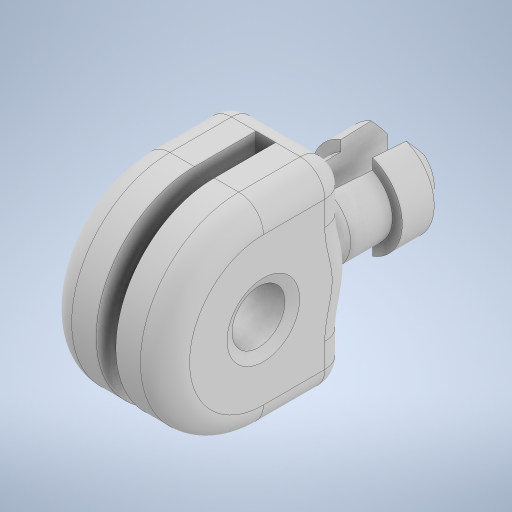
# Autodesk Inventor part: flipper_robot_v2_servo_flipper_adapter
Saved by Autodesk Inventor 2023.1 (Build 271208000, 208)
## iProperties
Created: 2025-10-28
Part Number: flipper_robot_v2_servo_flipper_adapter
Material: Generic
Document SubType Name: Modeling
Designer: Lars
Density: 1 g/cm^3
Appearance: Default
Author: Lars
Autodesk Inventor part; units mm, degrees
ref_plane "YZ Plane" through (0, 0, 0) normal (1, 0, 0) x (0, 1, 0)
ref_plane "XZ Plane" through (0, 0, 0) normal (0, 1, 0) x (-1, 0, 0)
sketch "Base Profile" plane through (0, 0, 0) normal (1, 0, 0) x (0, 1, 0)
  arc A0 (4, 0) -> (-4, 0) centre (0, 0) ccw
  line L0 (4, 0) -> (-4, 0) construction
  line L1 (-4, 0) -> (-4, -3.5)
  line L2 (-4, -3.5) -> (4, -3.5)
  line L3 (4, -3.5) -> (4, 0)
  circle A1 centre (0, 0) radius 1.075
  dimension "d0" = 8
  dimension "d1" = 3.5
  dimension "d2" = 2.15
  constraints: 8 end point, 2 centre point, 2 coincident, 2 parallel, 2 point on circle, 2 tangent, 1 horizontal, 1 perpendicular
  measures "d0" diameter of A0
  measures "d1" distance of L2.end L0.start
  measures "d2" diameter of A1
extrude "Clip Base" add sketch "Base Profile" along normal blind 4.8
ref_plane "Work Plane (Slot Cut)" through (0, 0, 4) normal (0, 0, -1) x (-1, 0, 0)
sketch "Fin Slot Layout" plane through (0, 0, 4) normal (0, 0, -1) x (-1, 0, 0)
  line L0 (0, -4) -> (-4.8, -4) projected
  line L1 (0, 4) -> (-4.8, 4) projected
  line L2 (-2.8, -4) -> (-2, -4)
  line L3 (-2, -4) -> (-2, 4)
  line L4 (-2, 4) -> (-2.8, 4)
  line L5 (-2.8, 4) -> (-2.8, -4)
  point P0 (0, 0)
  point P1 (-2.4, -4)
  dimension "d8" = 0.8
  constraints: 8 end point, 2 midpoint, 2 parallel, 2 point on line, 1 horizontal, 1 perpendicular
  measures "d8" distance between parallel lines of L3 L5
extrude "Fin Slot Cut" cut sketch "Fin Slot Layout" along normal blind 6.5
sketch "Shaft Profile" plane through (0, -4, -3.5) normal (0, 0, -1) x (-1, 0, 0)
  line L0 (0, 0) -> (0, 8) construction
  line L1 (0, 8) -> (-4.8, 8) construction
  line L2 (-4.8, 0) -> (-4.8, 8) construction
  line L3 (0, 0) -> (-4.8, 0) construction
  circle A0 centre (-2.4, 4) radius 1.45
  line L4 (-2.4, 8) -> (-2.4, 0) construction
  point P0 (0, 4)
  point P1 (-2.4, 4)
  dimension "d11" = 2.9
  constraints: 3 midpoint, 2 end point, 1 centre point, 1 coincident, 1 vertical
  measures "d11" diameter of A0
extrude "Snap Shaft" add sketch "Shaft Profile" along normal blind 4.7
sketch "Lip Profile" plane through (2.4, 0, -8.2) normal (0, 0, -1) x (-1, 0, 0)
  circle A0 centre (0, 0) radius 1.45 projected
  circle A1 centre (0, 0) radius 1.85
  point P0 (2.4, 0)
  dimension "d14" = 3.7
  constraints: 1 centre point, 1 coincident
  measures "d14" diameter of A1
extrude "Snap Lip" add sketch "Lip Profile" against normal blind 2
sketch "Upper Flex Profile" plane through (2.4, 0, -8.2) normal (0, 0, -1) x (-1, 0, 0)
  circle A0 centre (0, 0) radius 1.85 construction
  line L0 (-0.75, 1.85) -> (0.75, 1.85)
  line L1 (0.75, 1.85) -> (0.75, -1.85)
  line L2 (0.75, -1.85) -> (-0.75, -1.85)
  line L3 (-0.75, -1.85) -> (-0.75, 1.85)
  point P0 (2.4, 0)
  point P1 (0, 1.85)
  point P2 (0, -1.85)
  dimension "d18" = 1.5
  constraints: 8 end point, 2 midpoint, 2 parallel, 2 point on circle, 1 horizontal, 1 perpendicular, 1 tangent
  measures "d18" distance of L1.end L2.end
sketch "Lower Flex Profile" plane through (0, -4, -3.5) normal (0, 0, -1) x (-1, 0, 0)
  line L0 (-3.15, 5.85) -> (-1.65, 5.85) construction
  line L1 (-3.15, 2.15) -> (-3.15, 5.85) construction
  line L2 (-1.65, 2.15) -> (-3.15, 2.15) construction
  line L3 (-1.65, 5.85) -> (-1.65, 2.15) construction
  line L4 (-2.9, 5.875) -> (-1.9, 5.875)
  line L5 (-1.9, 5.875) -> (-1.9, 2.125)
  line L6 (-1.9, 2.125) -> (-2.9, 2.125)
  line L7 (-2.9, 2.125) -> (-2.9, 5.875)
  line L8 (-2.4, 2.125) -> (-2.4, 5.875) construction
  point P0 (0, 4)
  point P1 (-2.4, 4)
  point P2 (-2.4, 4)
  dimension "d20" = 1
  dimension "d21" = 3.75
  constraints: 10 end point, 3 midpoint, 2 parallel, 1 coincident, 1 horizontal, 1 perpendicular
  measures "d20" distance between parallel lines of L5 L7
  measures "d21" distance of L6.end L4.start
loft "Snap Flex Cut" cut profiles "Upper Flex Profile", "Lower Flex Profile"
chamfer "Entry Chamfer (Snap Tip)" distance 0.7 angle 45 2 edges at (4.25, 0, -8.2) (0.55, 0, -8.2)
fillet "Body Fillets (Clip Base)" radius 1 12 edges at (3.85, 0, -3.5) (0.95, 0, -3.5) (0, 0, -3.5) (4.8, 0, -3.5) (2.4, -4, -3.5) (2.4, 4, -3.5) (4.8, -4, -1.75) (4.8, 4, -1.75) (4.8, 0, 4) (0, -4, -1.75) (0, 4, -1.75) (0, 0, 4)
sketch "Hex Slot Profile" plane through (0, 0, 0) normal (-1, 0, 0) x (0, 0, 1)
  line L0 (-1.175, 2.0352) -> (1.175, 2.0352)
  line L1 (1.175, 2.0352) -> (2.35, 0)
  line L2 (2.35, 0) -> (1.175, -2.0352)
  line L3 (1.175, -2.0352) -> (-1.175, -2.0352)
  line L4 (-1.175, -2.0352) -> (-2.35, 0)
  line L5 (-2.35, 0) -> (-1.175, 2.0352)
  line L6 (0, 0) -> (-2.35, 0) construction
  dimension "d31" = 2.35
  constraints: 14 end point, 1 coincident, 1 horizontal, 13 other
  measures "d31" distance of L6.start L4.end
extrude "Hex Nut Slot" cut sketch "Hex Slot Profile" against normal blind 1
chamfer "Screw Head Chamfer (Outer Face)" distance 0.4 distance2 0.2 1 edges at (4.8, -1.075, 0)
equation "\"d21\" = d19"
equation "\"d19\" = 3.75"
body "Solid1"
